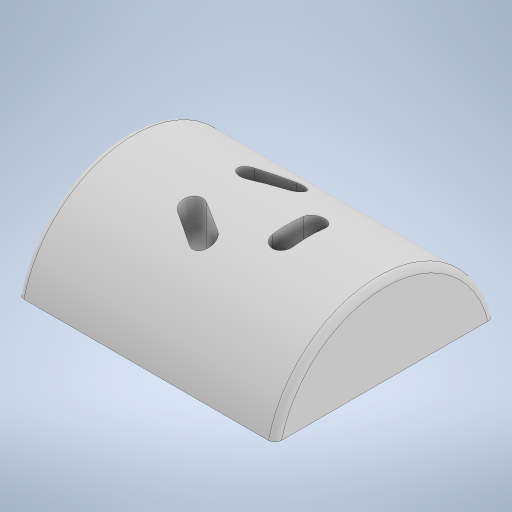
# Autodesk Inventor part: semicylinder_2
Saved by Autodesk Inventor 2024.2 (Build 282272000, 272)
## iProperties
Created: 2024-06-17
Part Number: semicylinder_2
Material: Ogólny
Document SubType Name: Modeling
Designer: Konrad
Density: 1 g/cm^3
Appearance: Domyślna
Author: Konrad
Autodesk Inventor part; units mm, degrees
ref_plane "YZ Plane" through (0, 0, 0) normal (1, 0, 0) x (0, 1, 0)
ref_plane "XZ Plane" through (0, 0, 0) normal (0, 1, 0) x (-1, 0, 0)
ref_plane "XY Plane" through (0, 0, 0) normal (0, 0, 1) x (1, 0, 0)
sketch "Szkic1" plane through (0, 0, 0) normal (0, 1, 0) x (-1, 0, 0)
  circle A0 centre (0, 0) radius 14.1 construction
  line L0 (0, 0) -> (-14.1, 0) construction
  circle A1 centre (0, 0) radius 22.5 construction
  circle A2 centre (-13.2497, 4.8225) radius 1.75
  circle A3 centre (-13.2497, -4.8225) radius 1.75
  circle A4 centre (2.4484, 13.8858) radius 1.75
  circle A5 centre (10.8012, 9.0633) radius 1.75
  circle A6 centre (10.8012, -9.0633) radius 1.75
  circle A7 centre (2.4484, -13.8858) radius 1.75
  circle A8 centre (0, 0) radius 35
  circle A9 centre (-13.2497, 4.8225) radius 3.25
  circle A10 centre (-13.2497, -4.8225) radius 3.25
  circle A11 centre (2.4484, -13.8858) radius 3.25
  circle A12 centre (10.8012, -9.0633) radius 3.25
  circle A13 centre (10.8012, 9.0633) radius 3.25
  circle A14 centre (2.4484, 13.8858) radius 3.25
  line L1 (12.4262, 11.8779) -> (4.0734, 16.7004)
  line L2 (9.1762, 6.2487) -> (0.8234, 11.0712)
  line L3 (-9.9997, 4.8225) -> (-9.9997, -4.8225)
  line L4 (12.4262, -11.8779) -> (4.0734, -16.7004)
  line L5 (9.1762, -6.2487) -> (0.8234, -11.0712)
  line L6 (-16.4997, -4.8225) -> (-16.4997, 4.8225)
  line L7 (-40, 35) -> (40, 35)
  line L8 (40, 35) -> (40, -35)
  line L9 (40, -35) -> (-40, -35)
  line L10 (-40, -35) -> (-40, 35)
  line L11 (-40, 35) -> (40, -35) construction
  line L12 (40, 35) -> (-40, -35) construction
  line L13 (0, -35) -> (0, 35)
  line L14 (40, 0) -> (-40, 0)
  line L15 (56, 0) -> (-56, 0) projected
  point P0 (0, -35)
  point P1 (0, 35)
  point P2 (35, 0)
  point P3 (-35, 0)
  dimension "d0" = 28.2
  dimension "d1" = 3.5
  dimension "d2" = 40
  dimension "d5" = 360
  dimension "d7" = 45
  dimension "d8" = 70
  dimension "d12" = 6.5
  dimension "d15" = 360
  dimension "d27" = 80
  dimension "d28" = 70
  constraints: 30 end point, 15 centre point, 15 point on circle, 12 tangent, 6 midpoint, 5 coincident, 2 equal radius, 2 horizontal, 2 parallel, 1 perpendicular, 1 symmetric about line, 26 other
  measures "d0" diameter of A0
  measures "d1" diameter of A2
  measures "d7" diameter of A1
  measures "d8" diameter of A8
  measures "d12" diameter of A9
  measures "d27" distance of L8.end L9.end
  measures "d28" distance of L7.end L8.end
revolve "Obrót2" add sketch "Szkic1" angle 180 about axis through (-10, 0, 0) along (-1, 0, 0) contours A2 | A4 | A5 | L14 L13 A14 L2 A13 L1 A8 | A8 L7 L8 L14 | L13 A14 L14 L3 A9 L6 A8 | A8 L14 L10 L7 | L13 A14 | A14 L13 | L14 L6 A9 L3 | L1 A13 L2 A14 | A9 | A13
extrude "Wyciągnięcie proste1" cut sketch "Szkic1" along normal through all contours A2 | A3 | A4 | A5 | A6 | A7 | L13 A14 | A14 L13 | L13 A11 | A11 L13 | L14 L6 A9 L3 | L3 A10 L6 L14 | L1 A13 L2 A14 | A11 L5 A12 L4 | A9 | A10 | A13 | A12
extrude "Wyciągnięcie proste2" add sketch "Szkic1" along normal blind 17.85 contours L13 A14 | A14 L13 | L13 A11 | A11 L13 | L14 L6 A9 L3 | L3 A10 L6 L14 | L1 A13 L2 A14 | A11 L5 A12 L4 | A9 | A10 | A13 | A12
extrude "Wyciągnięcie proste3" cut sketch "Szkic1" along normal blind 7.85 contours A2 | A3 | A4 | A5 | A6 | A7 | L14 L13 A14 L2 A13 L1 A8 | L14 L8 L9 A8 | A8 L7 L8 L14 | A8 L13 A11 L4 A12 L5 L14 | L13 A14 L14 L3 A9 L6 A8 | A8 L14 L10 L7 | L9 L10 L14 A8 | A8 L14 L6 A10 L3 L13 A11 | L13 A14 | A14 L13 | L13 A11 | A11 L13 | L14 L6 A9 L3 | L3 A10 L6 L14 | L1 A13 L2 A14 | A11 L5 A12 L4 | A9 | A10 | A13 | A12
fillet "Zaokrąglenie1" radius 2 2 edges at (-40, 35, 0) (40, 35, 0)
